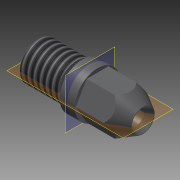
# Autodesk Inventor part: D-046
Saved by Autodesk Inventor 2015 (Build 190159000, 159)
## iProperties
Company: MARCHA TECHNOLOGY SL
Created: 2014-05-13
Part Number: D-046
Document SubType Name: Modeling
Designer: O.Martin
Density: 1 g/cm^3
Description: HOTEND ONE BODY TAPON
Stock Number: 28658
Project: HOTEND PROTOTIPO
Material: Generic
Appearance: Gray
Author: O.Martin
Autodesk Inventor part; units mm, degrees
ref_plane "YZ Plane" through (0, 0, 0) normal (1, 0, 0) x (0, 1, 0)
ref_plane "XZ Plane" through (0, 0, 0) normal (0, 1, 0) x (-1, 0, 0)
sketch "Boceto1" plane through (0, 0, 0) normal (0, 0, 1) x (1, 0, 0)
  line L0 (0, 0) -> (14, 0)
  line L1 (14, 0) -> (14, -1.5566)
  line L2 (14, -1.5566) -> (11.5, -3)
  line L3 (11.5, -3) -> (6, -3)
  line L4 (13.134, -1) -> (0, -1)
  line L5 (13.134, -1) -> (14, -1.5)
  line L6 (6, -2.0095) -> (6, -3)
  line L7 (0, -2.5) -> (0, -1)
  line L8 (0, -2.5) -> (5.25, -2.5)
  line L9 (5.25, -2.5) -> (5.25, -2.0095)
  line L10 (5.25, -2.0095) -> (6, -2.0095)
  dimension "d5" = 6
  dimension "d6" = 2.5
  dimension "d7" = 30
  dimension "d37" = 2
  dimension "d40" = 30
  dimension "d64" = 8
  dimension "d88" = 14
  dimension "d89" = 5
  dimension "d90" = 4.019
  dimension "d91" = 0.75
  dimension "d102" = 3
  constraints: 22 end point, 5 perpendicular, 1 coincident, 1 horizontal, 1 parallel, 1 point on line, 1 vertical, 1 vertical alignment
  measures "d5" diameter of L3 L0
  measures "d6" horizontal distance of L1.end L2.end
  measures "d7" angle of L2 L3
  measures "d37" diameter of L4 L0
  measures "d40" angle of L4 L5
  measures "d64" distance between parallel lines of L1 L6
  measures "d88" distance between parallel lines of L1 L7
  measures "d89" diameter of L8 L0
  measures "d90" diameter of L10 L0
  measures "d91" distance of L9.end L6.start
  measures "d102" diameter of L5.end L0
revolve "Revolución2" add sketch "Boceto1" angle 360 about axis through (0, 0, 0) along (1, 0, 0)
sketch "Boceto4" plane through (7, 0, 0) normal (-1, 0, 0) x (0, 0, 1)
  circle A0 centre (0, 0) radius 3 projected
  line L0 (1.6583, 2.5) -> (-1.6583, 2.5)
  line L1 (1.6583, -2.5) -> (-1.6583, -2.5)
  dimension "d99" = 5
  constraints: 4 end point, 4 point on circle, 2 parallel, 1 horizontal
  measures "d99" distance between parallel lines of L1 L0
sketch "Boceto2" plane through (4, 0, 0) normal (-1, 0, 0) x (0, 0, 1)
  circle A0 centre (0, 0) radius 2.5 projected
  line L0 (-6, 7) -> (13, 7)
  line L1 (13, 7) -> (13, -12)
  line L2 (13, -12) -> (-6, -12)
  line L3 (-6, -12) -> (-6, 7)
  dimension "d27" = 19
  dimension "d28" = 19
  dimension "d29" = 6
  dimension "d30" = 7
  constraints: 8 end point, 2 parallel, 1 horizontal, 1 perpendicular
  measures "d27" distance of L0.start L0.end
  measures "d28" distance of L0.end L1.end
  measures "d29" distance from line of A0.centre L3
  measures "d30" distance from line of A0.centre L0
thread "Rosca2" size "M5x0.8" class "6g" standard "ANSI Metric M Profile" full length
chamfer "Chaflán1" distance 0.25 angle 45 1 edges at (0, 2.5, 0)
ref_plane "Plano de trabajo1" through (7, 0, 0) normal (-1, 0, 0) x (0, 0, 1)
sketch "Boceto5" plane through (6, 0, 0) normal (-1, 0, 0) x (0, 0, 1)
  circle A0 centre (0, 0) radius 3 projected
  line L0 (0, 2.8868) -> (2.5, 1.4434)
  line L1 (2.5, 1.4434) -> (2.5, -1.4434)
  line L2 (2.5, -1.4434) -> (0, -2.8868)
  line L3 (0, -2.8868) -> (-2.5, -1.4434)
  line L4 (-2.5, -1.4434) -> (-2.5, 1.4434)
  line L5 (-2.5, 1.4434) -> (0, 2.8868)
  dimension "d103" = 5
  constraints: 12 end point, 1 coincident, 1 vertical, 13 other
  measures "d103" distance between parallel lines of L1 L4
extrude "Extrusión4" cut sketch "Boceto5" against normal through all
sketch "Boceto6" plane through (6, -1.4434, -2.5) normal (-1, 0, 0) x (0, 0, 1)
  line L0 (2.5, 4.3301) -> (0, 2.8868) projected
  line L1 (0, 2.8868) -> (0, 0) projected
  line L2 (0, 0) -> (2.5, -1.4434) projected
  line L3 (2.5, -1.4434) -> (5, 0) projected
  line L4 (5, 0) -> (5, 2.8868) projected
  line L5 (5, 2.8868) -> (2.5, 4.3301) projected
  circle A0 centre (2.5, 1.4434) radius 2.0095 projected
  circle A1 centre (2.5, 1.4434) radius 3
  dimension "d106" = 6
  constraints: 1 centre point, 1 coincident
  measures "d106" diameter of A1
extrude "Extrusión5" add sketch "Boceto6" against normal blind 2 contours A1
sketch "Boceto3" plane through (4, -7.4833, 13) normal (0, 0, 1) x (1, 0, 0)
  arc A0 (7.9608, 0) -> (2.0392, 0) centre (5, 0.4833) ccw projected
  point P0 (5, 7.4833)
  dimension "d41" = 7
  constraints: 1 vertical alignment
  measures "d41" distance of A0.centre point (5, 7.483)
body "Solid1"
